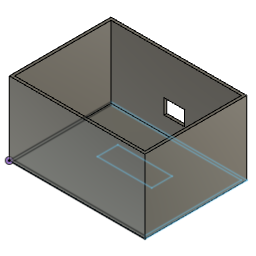
alarm_front v1 (Autodesk Fusion 360 design; units mm, degrees)
Autodesk Fusion 360 part; units mm, degrees
sketch "Sketch1" plane through (0, 0, 0) normal (0, 0, 1) x (1, 0, 0)
  line L0 (0, 0) -> (100, 0)
  line L1 (100, 0) -> (100, 75)
  line L2 (100, 75) -> (0, 75)
  line L3 (0, 75) -> (0, 0)
  line L4 (2, 2) -> (98, 2)
  line L5 (98, 2) -> (98, 73)
  line L6 (98, 73) -> (2, 73)
  line L7 (2, 73) -> (2, 2)
  line L8 (30, 50) -> (70, 50)
  line L9 (70, 50) -> (70, 35)
  line L10 (70, 35) -> (30, 35)
  line L11 (30, 35) -> (30, 50)
  dimension "d1" = -2
  constraint horizontal L0
  constraint vertical L1
  constraint horizontal L2
  constraint vertical L3
  constraint coincident L0.start L3.end
  constraint horizontal L8
  constraint vertical L9
  constraint horizontal L10
  constraint vertical L11
extrude "Extrude1" add sketch "Sketch1" along normal blind 1 contours L4 L5 L6 L7
extrude "Extrude2" add sketch "Sketch1" along normal blind 4 contours L0 L1 L2 L3
extrude "Extrude3" add 1 faces at (34, 0.6667, 4) along direction (0, 0, 1) blind 50
sketch "Sketch2" plane through (0, 75, 0) normal (0, 1, 0) x (-1, 0, 0)
  line L0 (-100, 0) -> (0, 0)
  line L1 (0, 0) -> (0, 54)
  line L2 (0, 54) -> (-100, 54)
  line L3 (-100, 54) -> (-100, 0)
  line L4 (-56.0994, 24.0994) -> (-41.0994, 24.0994)
  line L5 (-41.0994, 24.0994) -> (-41.0994, 13.0994)
  line L6 (-41.0994, 13.0994) -> (-56.0994, 13.0994)
  line L7 (-56.0994, 13.0994) -> (-56.0994, 24.0994)
  dimension "d8" = 15
  dimension "d9" = 11
  constraint horizontal L4
  constraint vertical L5
  constraint horizontal L6
  constraint vertical L7
  measures "d8" distance of L4.start L4.end
  measures "d9" distance of L4.start L6.end
extrude "Extrude4" cut sketch "Sketch2" against normal blind 15 contours L4 L5 L6 L7
